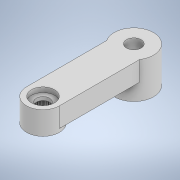
# Autodesk Inventor part: Поворотный рычаг для сервы
Saved by Autodesk Inventor 2020 (Build 240168000, 168)
## iProperties
Created: 2021-04-11
Part Number: Поворотный рычаг для сервы
Material: Типовые
Document SubType Name: Modeling
Designer: Антон
Density: 1 g/cm^3
Appearance: По умолчанию
Author: Антон
Autodesk Inventor part; units mm, degrees
ref_plane "YZ Plane" through (0, 0, 0) normal (1, 0, 0) x (0, 1, 0)
ref_plane "XZ Plane" through (0, 0, 0) normal (0, 1, 0) x (-1, 0, 0)
ref_plane "XY Plane" through (0, 0, 0) normal (0, 0, 1) x (1, 0, 0)
sketch "Эскиз1" plane through (0, 0, 0) normal (0, 1, 0) x (-1, 0, 0)
  circle A0 centre (0, 0) radius 3.35
  dimension "d0" = 6.7
  constraints: 1 centre point, 1 coincident
  measures "d0" diameter of A0
extrude "Выдавливание1" add sketch "Эскиз1" along normal blind 4.7
sketch "Эскиз2" plane through (0, 0, 0) normal (0, -1, 0) x (1, 0, 0)
  line L0 (0, 0) -> (2.375, 0)
  line L1 (2.375, 0) -> (2.4726, -0.0976)
  line L2 (2.375, 0) -> (2.4726, 0.0976)
  line L3 (2.4726, -0.0976) -> (2.4692, -0.1615)
  line L4 (2.362, 0.2483) -> (2.4692, 0.1614)
  line L5 (2.362, 0.2483) -> (2.4488, 0.3555)
  line L6 (2.4692, 0.1614) -> (2.4726, 0.0975)
  line L7 (2.3231, 0.4938) -> (2.4388, 0.4186)
  line L8 (2.3231, 0.4938) -> (2.3983, 0.6095)
  line L9 (2.4388, 0.4186) -> (2.4488, 0.3554)
  line L10 (2.2588, 0.7339) -> (2.3817, 0.6713)
  line L11 (2.2588, 0.7339) -> (2.3214, 0.8569)
  line L12 (2.3817, 0.6713) -> (2.3983, 0.6094)
  line L13 (2.1697, 0.966) -> (2.2985, 0.9165)
  line L14 (2.1697, 0.966) -> (2.2191, 1.0948)
  line L15 (2.2985, 0.9165) -> (2.3214, 0.8568)
  line L16 (2.0568, 1.1875) -> (2.1901, 1.1518)
  line L17 (2.0568, 1.1875) -> (2.0925, 1.3208)
  line L18 (2.1901, 1.1518) -> (2.2192, 1.0948)
  line L19 (1.9214, 1.396) -> (2.0577, 1.3744)
  line L20 (1.9214, 1.396) -> (1.943, 1.5323)
  line L21 (2.0577, 1.3744) -> (2.0926, 1.3207)
  line L22 (1.765, 1.5892) -> (1.9028, 1.582)
  line L23 (1.765, 1.5892) -> (1.7722, 1.727)
  line L24 (1.9028, 1.582) -> (1.9431, 1.5322)
  line L25 (1.5892, 1.765) -> (1.727, 1.7722)
  line L26 (1.5892, 1.765) -> (1.582, 1.9028)
  line L27 (1.727, 1.7722) -> (1.7723, 1.7269)
  line L28 (1.396, 1.9214) -> (1.5323, 1.943)
  line L29 (1.396, 1.9214) -> (1.3744, 2.0577)
  line L30 (1.5323, 1.943) -> (1.582, 1.9027)
  line L31 (1.1875, 2.0568) -> (1.3208, 2.0925)
  line L32 (1.1875, 2.0568) -> (1.1518, 2.1901)
  line L33 (1.3208, 2.0925) -> (1.3745, 2.0577)
  line L34 (0.966, 2.1697) -> (1.0948, 2.2191)
  line L35 (0.966, 2.1697) -> (0.9165, 2.2985)
  line L36 (1.0948, 2.2191) -> (1.1519, 2.1901)
  line L37 (0.7339, 2.2588) -> (0.8569, 2.3214)
  line L38 (0.7339, 2.2588) -> (0.6713, 2.3817)
  line L39 (0.8569, 2.3214) -> (0.9166, 2.2985)
  line L40 (0.4938, 2.3231) -> (0.6095, 2.3983)
  line L41 (0.4938, 2.3231) -> (0.4186, 2.4388)
  line L42 (0.6095, 2.3983) -> (0.6713, 2.3817)
  line L43 (0.2483, 2.362) -> (0.3555, 2.4488)
  line L44 (0.2483, 2.362) -> (0.1614, 2.4692)
  line L45 (0.3555, 2.4488) -> (0.4187, 2.4388)
  line L46 (0, 2.375) -> (0.0976, 2.4726)
  line L47 (0, 2.375) -> (-0.0976, 2.4726)
  line L48 (0.0976, 2.4726) -> (0.1615, 2.4692)
  line L49 (-0.2483, 2.362) -> (-0.1614, 2.4692)
  line L50 (-0.2483, 2.362) -> (-0.3555, 2.4488)
  line L51 (-0.1614, 2.4692) -> (-0.0975, 2.4726)
  line L52 (-0.4938, 2.3231) -> (-0.4186, 2.4388)
  line L53 (-0.4938, 2.3231) -> (-0.6095, 2.3983)
  line L54 (-0.4186, 2.4388) -> (-0.3554, 2.4488)
  line L55 (-0.7339, 2.2588) -> (-0.6713, 2.3817)
  line L56 (-0.7339, 2.2588) -> (-0.8569, 2.3214)
  line L57 (-0.6713, 2.3817) -> (-0.6094, 2.3983)
  line L58 (-0.966, 2.1697) -> (-0.9165, 2.2985)
  line L59 (-0.966, 2.1697) -> (-1.0948, 2.2191)
  line L60 (-0.9165, 2.2985) -> (-0.8568, 2.3214)
  line L61 (-1.1875, 2.0568) -> (-1.1518, 2.1901)
  line L62 (-1.1875, 2.0568) -> (-1.3208, 2.0925)
  line L63 (-1.1518, 2.1901) -> (-1.0948, 2.2192)
  line L64 (-1.396, 1.9214) -> (-1.3744, 2.0577)
  line L65 (-1.396, 1.9214) -> (-1.5323, 1.943)
  line L66 (-1.3744, 2.0577) -> (-1.3207, 2.0926)
  line L67 (-1.5892, 1.765) -> (-1.582, 1.9028)
  line L68 (-1.5892, 1.765) -> (-1.727, 1.7722)
  line L69 (-1.582, 1.9028) -> (-1.5322, 1.9431)
  line L70 (-1.765, 1.5892) -> (-1.7722, 1.727)
  line L71 (-1.765, 1.5892) -> (-1.9028, 1.582)
  line L72 (-1.7722, 1.727) -> (-1.7269, 1.7723)
  line L73 (-1.9214, 1.396) -> (-1.943, 1.5323)
  line L74 (-1.9214, 1.396) -> (-2.0577, 1.3744)
  line L75 (-1.943, 1.5323) -> (-1.9027, 1.582)
  line L76 (-2.0568, 1.1875) -> (-2.0925, 1.3208)
  line L77 (-2.0568, 1.1875) -> (-2.1901, 1.1518)
  line L78 (-2.0925, 1.3208) -> (-2.0577, 1.3745)
  line L79 (-2.1697, 0.966) -> (-2.2191, 1.0948)
  line L80 (-2.1697, 0.966) -> (-2.2985, 0.9165)
  line L81 (-2.2191, 1.0948) -> (-2.1901, 1.1519)
  line L82 (-2.2588, 0.7339) -> (-2.3214, 0.8569)
  line L83 (-2.2588, 0.7339) -> (-2.3817, 0.6713)
  line L84 (-2.3214, 0.8569) -> (-2.2985, 0.9166)
  line L85 (-2.3231, 0.4938) -> (-2.3983, 0.6095)
  line L86 (-2.3231, 0.4938) -> (-2.4388, 0.4186)
  line L87 (-2.3983, 0.6095) -> (-2.3817, 0.6713)
  line L88 (-2.362, 0.2483) -> (-2.4488, 0.3555)
  line L89 (-2.362, 0.2483) -> (-2.4692, 0.1614)
  line L90 (-2.4488, 0.3555) -> (-2.4388, 0.4187)
  line L91 (-2.375, 0) -> (-2.4726, 0.0976)
  line L92 (-2.375, 0) -> (-2.4726, -0.0976)
  line L93 (-2.4726, 0.0976) -> (-2.4692, 0.1615)
  line L94 (-2.362, -0.2483) -> (-2.4692, -0.1614)
  line L95 (-2.362, -0.2483) -> (-2.4488, -0.3555)
  line L96 (-2.4692, -0.1614) -> (-2.4726, -0.0975)
  line L97 (-2.3231, -0.4938) -> (-2.4388, -0.4186)
  line L98 (-2.3231, -0.4938) -> (-2.3983, -0.6095)
  line L99 (-2.4388, -0.4186) -> (-2.4488, -0.3554)
  line L100 (-2.2588, -0.7339) -> (-2.3817, -0.6713)
  line L101 (-2.2588, -0.7339) -> (-2.3214, -0.8569)
  line L102 (-2.3817, -0.6713) -> (-2.3983, -0.6094)
  line L103 (-2.1697, -0.966) -> (-2.2985, -0.9165)
  line L104 (-2.1697, -0.966) -> (-2.2191, -1.0948)
  line L105 (-2.2985, -0.9165) -> (-2.3214, -0.8568)
  line L106 (-2.0568, -1.1875) -> (-2.1901, -1.1518)
  line L107 (-2.0568, -1.1875) -> (-2.0925, -1.3208)
  line L108 (-2.1901, -1.1518) -> (-2.2192, -1.0948)
  line L109 (-1.9214, -1.396) -> (-2.0577, -1.3744)
  line L110 (-1.9214, -1.396) -> (-1.943, -1.5323)
  line L111 (-2.0577, -1.3744) -> (-2.0926, -1.3207)
  line L112 (-1.765, -1.5892) -> (-1.9028, -1.582)
  line L113 (-1.765, -1.5892) -> (-1.7722, -1.727)
  line L114 (-1.9028, -1.582) -> (-1.9431, -1.5322)
  line L115 (-1.5892, -1.765) -> (-1.727, -1.7722)
  line L116 (-1.5892, -1.765) -> (-1.582, -1.9028)
  line L117 (-1.727, -1.7722) -> (-1.7723, -1.7269)
  line L118 (-1.396, -1.9214) -> (-1.5323, -1.943)
  line L119 (-1.396, -1.9214) -> (-1.3744, -2.0577)
  line L120 (-1.5323, -1.943) -> (-1.582, -1.9027)
  line L121 (-1.1875, -2.0568) -> (-1.3208, -2.0925)
  line L122 (-1.1875, -2.0568) -> (-1.1518, -2.1901)
  line L123 (-1.3208, -2.0925) -> (-1.3745, -2.0577)
  line L124 (-0.966, -2.1697) -> (-1.0948, -2.2191)
  line L125 (-0.966, -2.1697) -> (-0.9165, -2.2985)
  line L126 (-1.0948, -2.2191) -> (-1.1519, -2.1901)
  line L127 (-0.7339, -2.2588) -> (-0.8569, -2.3214)
  line L128 (-0.7339, -2.2588) -> (-0.6713, -2.3817)
  line L129 (-0.8569, -2.3214) -> (-0.9166, -2.2985)
  line L130 (-0.4938, -2.3231) -> (-0.6095, -2.3983)
  line L131 (-0.4938, -2.3231) -> (-0.4186, -2.4388)
  line L132 (-0.6095, -2.3983) -> (-0.6713, -2.3817)
  line L133 (-0.2483, -2.362) -> (-0.3555, -2.4488)
  line L134 (-0.2483, -2.362) -> (-0.1614, -2.4692)
  line L135 (-0.3555, -2.4488) -> (-0.4187, -2.4388)
  line L136 (0, -2.375) -> (-0.0976, -2.4726)
  line L137 (0, -2.375) -> (0.0976, -2.4726)
  line L138 (-0.0976, -2.4726) -> (-0.1615, -2.4692)
  line L139 (0.2483, -2.362) -> (0.1614, -2.4692)
  line L140 (0.2483, -2.362) -> (0.3555, -2.4488)
  line L141 (0.1614, -2.4692) -> (0.0975, -2.4726)
  line L142 (0.4938, -2.3231) -> (0.4186, -2.4388)
  line L143 (0.4938, -2.3231) -> (0.6095, -2.3983)
  line L144 (0.4186, -2.4388) -> (0.3554, -2.4488)
  line L145 (0.7339, -2.2588) -> (0.6713, -2.3817)
  line L146 (0.7339, -2.2588) -> (0.8569, -2.3214)
  line L147 (0.6713, -2.3817) -> (0.6094, -2.3983)
  line L148 (0.966, -2.1697) -> (0.9165, -2.2985)
  line L149 (0.966, -2.1697) -> (1.0948, -2.2191)
  line L150 (0.9165, -2.2985) -> (0.8568, -2.3214)
  line L151 (1.1875, -2.0568) -> (1.1518, -2.1901)
  line L152 (1.1875, -2.0568) -> (1.3208, -2.0925)
  line L153 (1.1518, -2.1901) -> (1.0948, -2.2192)
  line L154 (1.396, -1.9214) -> (1.3744, -2.0577)
  line L155 (1.396, -1.9214) -> (1.5323, -1.943)
  line L156 (1.3744, -2.0577) -> (1.3207, -2.0926)
  line L157 (1.5892, -1.765) -> (1.582, -1.9028)
  line L158 (1.5892, -1.765) -> (1.727, -1.7722)
  line L159 (1.582, -1.9028) -> (1.5322, -1.9431)
  line L160 (1.765, -1.5892) -> (1.7722, -1.727)
  line L161 (1.765, -1.5892) -> (1.9028, -1.582)
  line L162 (1.7722, -1.727) -> (1.7269, -1.7723)
  line L163 (1.9214, -1.396) -> (1.943, -1.5323)
  line L164 (1.9214, -1.396) -> (2.0577, -1.3744)
  line L165 (1.943, -1.5323) -> (1.9027, -1.582)
  line L166 (2.0568, -1.1875) -> (2.0925, -1.3208)
  line L167 (2.0568, -1.1875) -> (2.1901, -1.1518)
  line L168 (2.0925, -1.3208) -> (2.0577, -1.3745)
  line L169 (2.1697, -0.966) -> (2.2191, -1.0948)
  line L170 (2.1697, -0.966) -> (2.2985, -0.9165)
  line L171 (2.2191, -1.0948) -> (2.1901, -1.1519)
  line L172 (2.2588, -0.7339) -> (2.3214, -0.8569)
  line L173 (2.2588, -0.7339) -> (2.3817, -0.6713)
  line L174 (2.3214, -0.8569) -> (2.2985, -0.9166)
  line L175 (2.3231, -0.4938) -> (2.3983, -0.6095)
  line L176 (2.3231, -0.4938) -> (2.4388, -0.4186)
  line L177 (2.3983, -0.6095) -> (2.3817, -0.6713)
  line L178 (2.362, -0.2483) -> (2.4488, -0.3555)
  line L179 (2.362, -0.2483) -> (2.4692, -0.1614)
  line L180 (2.4488, -0.3555) -> (2.4388, -0.4187)
  dimension "d3" = 2.375
  dimension "d4" = 0.138
  dimension "d5" = 0.138
  dimension "d6" = 135
  dimension "d7" = 135
  dimension "d9" = 0.064
  dimension "d10" = 132
  dimension "d13" = 360
  constraints: 362 end point, 1 horizontal, 421 other
  measures "d3" distance of L0.start L0.end
  measures "d4" distance of L0.end L1.end
  measures "d5" distance of L0.end L2.end
  measures "d6" angle of L0 L2
  measures "d7" angle of L0 L1
  measures "d9" distance of L1.end L3.end
  measures "d10" angle of L1 L3
extrude "Выдавливание2" cut sketch "Эскиз2" against normal blind 3
sketch "Эскиз3" plane through (0, 4.7, 0) normal (0, 1, 0) x (1, 0, 0)
  circle A0 centre (0, 0) radius 2.35
  dimension "d17" = 4.7
  constraints: 1 centre point, 1 coincident
  measures "d17" diameter of A0
extrude "Выдавливание3" cut sketch "Эскиз3" against normal blind 1
sketch "Эскиз4" plane through (0, 3.7, 0) normal (0, 1, 0) x (1, 0, 0)
  point P0 (0, 0)
  point P1 (0, 0)
  constraints: 1 coincident
hole "Отверстие1" at (0, 3.7, 0) direction (0, -1, 0) diameter 2.7 end through all
sketch "Эскиз5" plane through (0, 4.7, 0) normal (0, 1, 0) x (1, 0, 0)
  circle A0 centre (0, 0) radius 3.35 projected
  line L0 (-3.35, 0) -> (3.35, 0)
  line L1 (3.35, 0) -> (3.35, 18.5)
  line L2 (3.35, 18.5) -> (-3.35, 18.5)
  line L3 (-3.35, 18.5) -> (-3.35, 0)
  dimension "d27" = 18.5
  constraints: 8 end point, 2 parallel, 1 horizontal, 1 perpendicular, 2 other
  measures "d27" distance of L1.end L0.end
extrude "Выдавливание4" add sketch "Эскиз5" against normal blind 4 contours A0 L3 L2 L1
sketch "Эскиз6" plane through (0, 4.7, 0) normal (0, 1, 0) x (1, 0, 0)
  line L0 (-3.35, 18.5) -> (3.35, 18.5) projected
  circle A0 centre (0, 18.5) radius 4
  point P0 (0, 0)
  dimension "d30" = 8
  constraints: 1 centre point, 1 midpoint
  measures "d30" diameter of A0
extrude "Выдавливание5" add sketch "Эскиз6" against normal blind 7.35
sketch "Эскиз7" plane through (0, -2.65, -18.5) normal (0, -1, 0) x (1, 0, 0)
  circle A0 centre (0, 0) radius 4 projected
  arc A1 (3.35, 2.1857) -> (-3.35, 2.1857) centre (0, 0) ccw projected
  circle A2 centre (0, 0) radius 2.5
  point P0 (0, 18.5)
  dimension "d33" = 5
  constraints: 1 centre point, 1 coincident
  measures "d33" diameter of A2
extrude "Выдавливание6" cut sketch "Эскиз7" against normal blind 2.5 contours A2
sketch "Эскиз8" plane through (0, 4.7, 0) normal (0, 1, 0) x (1, 0, 0)
  circle A0 centre (0, 18.5) radius 2.5 projected
  point P0 (0, 0)
hole "Отверстие2" at (0, 4.7, -18.5) direction (0, -1, 0) diameter 3 end through all
